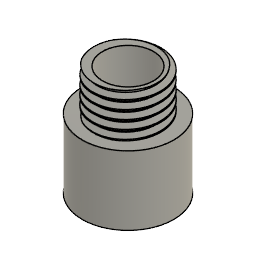
AG08 (Autodesk Fusion 360 archive; units mm, degrees)
design "Conector pvc"
part number: 2025-09-11-09-41-15-964
Autodesk Fusion 360 part; units mm, degrees
sketch "Boceto1" plane through (0, 0, 0) normal (0, 0, 1) x (1, 0, 0)
  circle A0 centre (0, 0) radius 13.3
  dimension "d1" = 26.6
  constraint coincident A0.centre origin
  measures "d1" diameter of A0
extrude "Extruir1" add sketch "Boceto1" along normal blind 20
sketch "Boceto2" plane through (0, 0, 20) normal (0, 0, 1) x (-1, 0, 0)
  circle A0 centre (0, 0) radius 13.3
  circle A1 centre (0, 0) radius 10.25
  circle A2 centre (0, 0) radius 7.4
  dimension "d5" = 20.5
  dimension "d6" = 14.8
  constraint coincident A0.centre A1.centre
  constraint concentric A1 A2
  measures "d5" diameter of A1
  measures "d6" diameter of A2
extrude "Extruir2" add sketch "Boceto2" along normal blind 11.9 contours A1
sketch "Boceto3" plane through (0, 0, 0) normal (0, 0, -1) x (1, 0, 0)
  circle A0 centre (0, 0) radius 13.3
  circle A1 centre (0, 0) radius 10.8
  dimension "d9" = 21.6
  constraint coincident A0.centre A1.centre
  measures "d9" diameter of A1
extrude "Extruir3" cut sketch "Boceto3" against normal blind 19 contours A1
extrude "Extruir4" cut 1 faces at (-1.5104, -2.2962, 20) along direction (0, 0, -1) blind 5
thread "Rosca1" "ISO Metric profile 20.0 M20x2.5 M20x2.5 6g" major diameter 19.7905 minor diameter 16.938 pitch 2.5 angle 60 modelled right hand crest width 0.36 on face at (-10.1991, 1.0206, 23.9667) crest through (-9.8953, 0, 19.375)
chamfer "Chaflán1" distance 2 angle 45 1 edges at (6.8992, 2.676, 19)

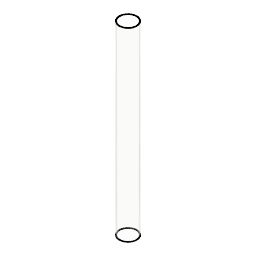
design "Tubo"
part number: 2025-09-05-15-36-02-729
Autodesk Fusion 360 part; units mm, degrees
sketch "Boceto1" plane through (0, 0, 0) normal (0, 0, 1) x (1, 0, 0)
  circle A0 centre (0, 0) radius 40.2
  dimension "d1" = 80.4
  constraint coincident A0.centre origin
  measures "d1" diameter of A0
extrude "Extruir1" add sketch "Boceto1" along normal blind 840
sketch "Boceto2" plane through (0, 0, 840) normal (0, 0, 1) x (-1, 0, 0)
  circle A0 centre (0, 0) radius 40.2
  circle A1 centre (0, 0) radius 37.3
  dimension "d4" = 74.6
  constraint coincident A0.centre A1.centre
  measures "d4" diameter of A1
extrude "Extruir2" cut sketch "Boceto2" against normal blind 880 contours A1
